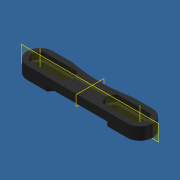
# Autodesk Inventor part: Shoulder_spanner
Saved by Autodesk Inventor 2016 (Build 200138000, 138)
## iProperties
Created: 2015-02-18
Part Number: Shoulder_spanner
Material: ABS-Kunststoff - Schwarz
Document SubType Name: Modeling
Designer: 4ndreas
Density: 1.06 g/cm^3
Appearance: Glatt - weiß(2)
Mass: 2.69052 g
Surface Area: 24.1446 cm^2
Volume: 2.53823 cm^3
Author: 4ndreas
Autodesk Inventor part; units mm, degrees
ref_plane "YZ Plane" through (0, 0, 0) normal (1, 0, 0) x (0, 1, 0)
ref_plane "XZ Plane" through (0, 0, 0) normal (0, 1, 0) x (-1, 0, 0)
ref_plane "XY Plane" through (0, 0, 0) normal (0, 0, 1) x (1, 0, 0)
sketch "Skizze1" plane through (0, 0, 0) normal (0, 0, 1) x (1, 0, 0)
  line L0 (-30.1531, -2.1) -> (-42.6531, -2.1) projected
  arc A0 (-42.6531, 2.1) -> (-42.6531, -2.1) centre (-42.6531, 0) ccw projected
  line L1 (-42.6531, 2.1) -> (-30.1531, 2.1) projected
  arc A1 (-30.1531, -2.1) -> (-30.1531, 2.1) centre (-30.1531, 0) ccw projected
  arc A2 (-7.1127, 2.1) -> (-7.1127, -2.1) centre (-7.1127, 0) ccw projected
  line L2 (-7.1127, 2.1) -> (5.3873, 2.1) projected
  arc A3 (5.3873, -2.1) -> (5.3873, 2.1) centre (5.3873, 0) ccw projected
  line L3 (5.3873, -2.1) -> (-7.1127, -2.1) projected
  circle A4 centre (-18.6329, -15.05) radius 14 projected
  circle A5 centre (-18.6329, 73.2719) radius 11.05 projected
  arc A6 (19.5363, 49.4369) -> (23.7773, 46.7885) centre (21.6568, 48.1127) ccw projected
  arc A7 (19.5363, 49.4369) -> (-57.3137, 50.2763) centre (-18.6329, 73.2719) ccw projected
  spline S0 degree 3 poles (-57.3137, 50.2763) (-57.1415, 49.9867) (-56.9966, 49.6783) (-56.7784, 49.0519) (-56.7017, 48.7303) (-56.6239, 48.0366) (-56.6345, 47.6574) (-56.7807, 47.0301) (-56.8829, 46.7742) (-57.1624, 46.3502) (-57.3235, 46.1805) (-57.5157, 46.0459) knots 0 0 0 0 0.100197 0.100197 0.197338 0.197338 0.308151 0.308151 0.389963 0.389963 0.460336 0.460336 0.460336 0.460336 projected
  line L4 (-57.5157, 46.0459) -> (-57.5426, 46.0271) projected
  ellipse E0 centre (-59.5705, 48.9232) end of major axis (-61.5984, 51.8193) minor radius 2.5 (-61.0744, 46.8387) -> (-57.5426, 46.0271) ccw projected
  arc A8 (23.7773, 46.7885) -> (-61.0744, 46.8387) centre (-18.6329, 73.2719) ccw projected
  line L5 (-0.8579, 86.6698) -> (-3.6329, 85.0676) projected
  line L6 (-3.6329, 85.0676) -> (-6.4079, 86.6698) projected
  line L7 (-6.4079, 86.6698) -> (-6.4079, 89.8741) projected
  line L8 (-6.4079, 89.8741) -> (-3.6329, 91.4762) projected
  line L9 (-3.6329, 91.4762) -> (-0.8579, 89.8741) projected
  line L10 (-0.8579, 89.8741) -> (-0.8579, 86.6698) projected
  line L11 (-6.4079, 59.8741) -> (-3.6329, 61.4762) projected
  line L12 (-3.6329, 61.4762) -> (-0.8579, 59.8741) projected
  line L13 (-0.8579, 59.8741) -> (-0.8579, 56.6698) projected
  line L14 (-0.8579, 56.6698) -> (-3.6329, 55.0676) projected
  line L15 (-3.6329, 55.0676) -> (-6.4079, 56.6698) projected
  line L16 (-6.4079, 56.6698) -> (-6.4079, 59.8741) projected
  line L17 (-36.4079, 59.8741) -> (-33.6329, 61.4762) projected
  line L18 (-33.6329, 61.4762) -> (-30.8579, 59.8741) projected
  line L19 (-30.8579, 59.8741) -> (-30.8579, 56.6698) projected
  line L20 (-30.8579, 56.6698) -> (-33.6329, 55.0676) projected
  line L21 (-33.6329, 55.0676) -> (-36.4079, 56.6698) projected
  line L22 (-36.4079, 56.6698) -> (-36.4079, 59.8741) projected
  line L23 (-30.8579, 86.6698) -> (-33.6329, 85.0676) projected
  line L24 (-33.6329, 85.0676) -> (-36.4079, 86.6698) projected
  line L25 (-36.4079, 86.6698) -> (-36.4079, 89.8741) projected
  line L26 (-36.4079, 89.8741) -> (-33.6329, 91.4762) projected
  line L27 (-33.6329, 91.4762) -> (-30.8579, 89.8741) projected
  line L28 (-30.8579, 89.8741) -> (-30.8579, 86.6698) projected
  line L29 (-21.6329, -35.1) -> (-21.6329, -48.7281) projected
  line L30 (-15.6329, -48.7281) -> (-21.6329, -48.7281) projected
  line L31 (-15.6329, -35.1) -> (-15.6329, -48.7281) projected
  line L32 (-3.5829, -35.1) -> (-15.6329, -35.1) projected
  arc A9 (-3.5829, -35.1) -> (1.4171, -30.1) centre (-3.5829, -30.1) ccw projected
  line L33 (1.4171, -22.1174) -> (1.4171, -30.1) projected
  spline S1 degree 3 poles (5.4171, -15.0509) (5.4147, -15.0534) (5.4123, -15.0559) (4.6387, -15.8583) (3.8622, -16.6655) (2.6723, -18.2412) (2.1512, -19.0655) (1.5603, -20.6885) (1.4171, -21.3977) (1.4171, -22.1174) knots 0 0 0 0 0.0012 0.0012 0.384075 0.384075 0.683828 0.683828 0.899728 0.899728 0.899728 0.899728 projected
  arc A10 (48.8863, -32.4077) -> (5.4171, -15.0509) centre (-18.6329, -138.3947) ccw projected
  spline S2 degree 3 poles (46.6689, -28.6102) (46.687, -28.6358) (46.7052, -28.6619) (47.5464, -29.8644) (48.2846, -31.1065) (48.8863, -32.4077) knots 0 0 0 0 0.009408 0.009408 0.428044 0.428044 0.428044 0.428044 projected
  spline S3 degree 3 poles (46.3671, 73.2719) (46.3671, 69.062) (45.5995, 65.0904) (43.0366, 57.3871) (41.3844, 53.8297) (36.5234, 43.9303) (33.0874, 37.527) (29.4142, 24.4534) (28.6107, 18.1121) (30.256, 4.2032) (32.4354, -3.9552) (40.4412, -19.2682) (43.5252, -24.1471) (46.6689, -28.6102) knots -13.775579 -13.775579 -13.775579 -13.775579 -11.916531 -11.916531 -10.206507 -10.206507 -7.199912 -7.199912 -4.876321 -4.876321 -2.796234 -2.796234 -1.753011 -1.753011 -1.753011 -1.753011 projected
  arc A11 (46.3671, 73.2719) -> (-83.6329, 73.2719) centre (-18.6329, 73.2719) ccw projected
  spline S4 degree 3 poles (-83.9347, -28.6102) (-82.7069, -26.8671) (-81.4925, -25.0666) (-75.3921, -15.5288) (-70.9948, -6.9499) (-66.4184, 9.431) (-66.0615, 15.8887) (-67.4531, 29.6924) (-70.2546, 36.5869) (-76.2635, 49.1483) (-79.4526, 54.8792) (-82.8508, 65.0165) (-83.6329, 69.0218) (-83.6329, 73.2719) knots -8.648216 -8.648216 -8.648216 -8.648216 -8.254246 -8.254246 -6.614154 -6.614154 -5.212744 -5.212744 -3.192896 -3.192896 -1.275036 -1.275036 0 0 0 0 projected
  spline S5 degree 3 poles (-86.1522, -32.4077) (-85.9485, -31.9672) (-85.7293, -31.5338) (-85.2658, -30.6848) (-85.0214, -30.2686) (-84.6343, -29.6497) (-84.4998, -29.4414) (-84.293, -29.1304) (-84.2227, -29.0263) (-84.116, -28.8704) (-84.0801, -28.8184) (-84.0259, -28.7403) (-84.0078, -28.7143) (-83.9711, -28.6619) (-83.9528, -28.6358) (-83.9347, -28.6102) knots 0.128552 0.128552 0.128552 0.128552 0.274044 0.274044 0.418651 0.418651 0.49297 0.49297 0.530648 0.530648 0.549617 0.549617 0.559135 0.559135 0.568808 0.568808 0.568808 0.568808 projected
  arc A12 (-42.6829, -15.0509) -> (-86.1522, -32.4077) centre (-18.6329, -138.3947) ccw projected
  spline S6 degree 3 poles (-38.6829, -22.1174) (-38.6829, -21.3977) (-38.8261, -20.6885) (-39.4171, -19.0655) (-39.9382, -18.2412) (-41.128, -16.6655) (-41.9045, -15.8583) (-42.6781, -15.0559) (-42.6805, -15.0534) (-42.6829, -15.0509) knots -0.001044 -0.001044 -0.001044 -0.001044 0.186915 0.186915 0.447875 0.447875 0.7812 0.7812 0.782245 0.782245 0.782245 0.782245 projected
  line L34 (-38.6829, -30.1) -> (-38.6829, -22.1174) projected
  arc A13 (-38.6829, -30.1) -> (-33.6829, -35.1) centre (-33.6829, -30.1) ccw projected
  line L35 (-21.6329, -35.1) -> (-33.6829, -35.1) projected
  arc A14 (11.642, 130.7909) -> (11.642, 15.753) centre (-18.6329, 73.2719) ccw projected
  spline S7 degree 3 poles (12.5639, 132.5424) (6.5678, 135.6985) (0.1274, 137.9264) (-13.2016, 140.3737) (-20.0134, 140.579) (-35.3971, 138.7033) (-43.7658, 135.9668) (-58.983, 127.4399) (-65.6862, 121.7311) (-76.5269, 108.0654) (-80.5608, 100.2392) (-85.4017, 83.481) (-86.1624, 74.7092) (-84.2786, 57.3678) (-81.6522, 48.964) (-73.3257, 33.6361) (-67.7054, 26.8586) (-54.1831, 15.8395) (-46.4105, 11.7032) (-29.7172, 6.6428) (-20.9562, 5.7671) (-3.5916, 7.4232) (4.846, 9.9391) (12.5639, 14.0014) knots -27.614157 -27.614157 -27.614157 -27.614157 -25.581379 -25.581379 -23.548602 -23.548602 -20.93209 -20.93209 -18.315579 -18.315579 -15.699068 -15.699068 -13.082556 -13.082556 -10.466045 -10.466045 -7.849534 -7.849534 -5.233023 -5.233023 -2.616511 -2.616511 0 0 0 0 projected
  line L36 (-42.6531, 0) -> (5.3873, 0) construction
  line L37 (-42.6531, -6.1) -> (5.3873, -6.1)
  line L38 (5.3873, 6.1) -> (-42.6531, 6.1)
  arc A15 (-42.6531, 6.1) -> (-42.6531, -6.1) centre (-42.6531, 0) ccw
  arc A16 (5.3873, -6.1) -> (5.3873, 6.1) centre (5.3873, 0) ccw
  arc A17 (-4.1788, -6.1) -> (-33.087, -6.1) centre (-18.6329, -40.2677) ccw
  arc A18 (-33.087, 6.1) -> (-4.1788, 6.1) centre (-18.6329, 74.9906) ccw
  line L39 (-18.6329, 6.1) -> (-18.6329, -6.1) construction
  line L40 (-30.1531, 4.6) -> (-7.1127, 4.6) construction
  line L41 (-7.1127, 4.6) -> (-7.1127, -3.1685) construction
  line L42 (-7.1127, -3.1685) -> (-30.1531, -3.1685) construction
  line L43 (-30.1531, -3.1685) -> (-30.1531, 4.6) construction
  line L44 (-33.087, 6.1) -> (-4.1788, 6.1) construction
  line L45 (-4.1788, 6.1) -> (-4.1788, -6.1) construction
  line L46 (-4.1788, -6.1) -> (-33.087, -6.1) construction
  line L47 (-33.087, -6.1) -> (-33.087, 6.1) construction
  point P0 (0, 0)
  point P1 (-3.5829, 0)
  point P2 (-18.6329, 0)
  dimension "d0" = 4
  dimension "d1" = 1.5
  constraints: 26 end point, 8 point on circle, 6 parallel, 6 tangent, 5 point on line, 4 centre point, 3 midpoint, 2 horizontal, 2 perpendicular, 2 symmetric about line, 2 other
  measures "d0" radial gap between concentric circles of A15 A0
  measures "d1" distance between parallel lines of L38 L40
extrude "Extrusion1" add sketch "Skizze1" along normal blind 6 contours A17 A4 | A4 A17 L37 A15 L38 A18 A16
sketch "Skizze2" plane through (0, 0, 6) normal (0, 0, 1) x (1, 0, 0)
  arc A0 (-42.6531, 2.1) -> (-42.6531, -2.1) centre (-42.6531, 0) ccw projected
  line L0 (-42.6531, 2.1) -> (-30.1531, 2.1) projected
  arc A1 (-30.1531, -2.1) -> (-30.1531, 2.1) centre (-30.1531, 0) ccw projected
  line L1 (-30.1531, -2.1) -> (-42.6531, -2.1) projected
  arc A2 (-4.1788, -6.1) -> (-33.087, -6.1) centre (-18.6329, -40.2677) ccw projected
  arc A3 (-33.087, 6.1) -> (-4.1788, 6.1) centre (-18.6329, 74.9906) ccw projected
  arc A4 (-42.6531, 6.1) -> (-42.6531, -6.1) centre (-42.6531, 0) ccw projected
  line L2 (-46.6946, 0) -> (-44.6739, 3.5)
  line L3 (-44.6739, 3.5) -> (-40.6324, 3.5)
  line L4 (-40.6324, 3.5) -> (-38.6117, 0)
  line L5 (-38.6117, 0) -> (-40.6324, -3.5)
  line L6 (-40.6324, -3.5) -> (-44.6739, -3.5)
  line L7 (-44.6739, -3.5) -> (-46.6946, 0)
  line L8 (-26.1117, 0) -> (-28.1324, -3.5)
  line L9 (-28.1324, -3.5) -> (-32.1739, -3.5)
  line L10 (-32.1739, -3.5) -> (-34.1946, 0)
  line L11 (-34.1946, 0) -> (-32.1739, 3.5)
  line L12 (-32.1739, 3.5) -> (-28.1324, 3.5)
  line L13 (-28.1324, 3.5) -> (-26.1117, 0)
  line L14 (-40.6324, 3.5) -> (-32.1739, 3.5)
  line L15 (-32.1739, 3.5) -> (-32.1739, -3.5)
  line L16 (-32.1739, -3.5) -> (-40.6324, -3.5)
  line L17 (-40.6324, -3.5) -> (-40.6324, 3.5)
  line L18 (-18.6329, 4.6) -> (-18.6329, -3.1685)
  point P0 (0, 0)
  dimension "d4" = 7
  constraints: 35 end point, 2 coincident, 2 parallel, 2 point on circle, 1 horizontal, 1 perpendicular, 26 other
  measures "d4" distance between parallel lines of L16 L14
extrude "Extrusion2" cut sketch "Skizze2" against normal blind 3
ref_plane "Arbeitsebene1" through (-18.6329, 4.6, 6) normal (-1, 0, 0) x (0, -1, 0)
mirror "Spiegeln1" about plane through (-18.6329, 4.6, 6) normal (-1, 0, 0) of "Extrusion2"
sketch "Skizze3" plane through (0, 0, 6) normal (0, 0, 1) x (1, 0, 0)
  arc A0 (-4.1788, -6.1) -> (-33.087, -6.1) centre (-18.6329, -40.2677) ccw projected
  line L0 (-4.1788, -6.1) -> (5.3873, -6.1) projected
  line L1 (-33.087, -6.1) -> (-4.1788, -6.1)
  point P0 (0, 0)
  constraints: 2 end point, 1 collinear
extrude "Extrusion3" add sketch "Skizze3" against normal up to surface (6 mm away)
sketch "Skizze4" plane through (0, 0, 0) normal (0, 0, -1) x (-1, 0, 0)
  circle A0 centre (18.6329, -15.05) radius 14 projected
  circle A1 centre (18.6329, -15.05) radius 17
  point P0 (0, 0)
  dimension "d15" = 34
  constraints: 1 centre point
  measures "d15" diameter of A1
extrude "Extrusion4" cut sketch "Skizze4" against normal blind 2 contours A0 | A1
ref_plane "Arbeitsebene2" through (5.3873, 0, 0) normal (0, -1, 0) x (0, 0, 1)
